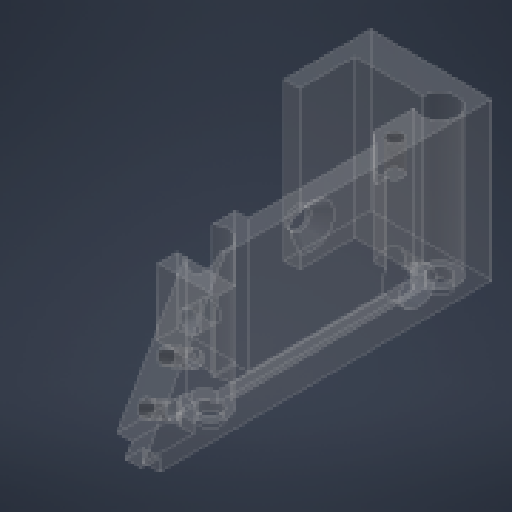
# Autodesk Inventor part: Lewybok
Saved by Autodesk Inventor 2023 (Build 270158000, 158)
## iProperties
Created: 2022-01-30
Part Number: Lewybok
Material: Tworzywo sztuczne PMMA
Document SubType Name: Modeling
Designer: Michał
Density: 1.188 g/cm^3
Appearance: Poliwęglan — przezroczysty
Mass: 9.32104 g
Surface Area: 57.3385 cm^2
Volume: 7.84599 cm^3
Author: Michał
Autodesk Inventor part; units mm, degrees
ref_plane "YZ Plane" through (0, 0, 0) normal (1, 0, 0) x (0, 1, 0)
ref_plane "XZ Plane" through (0, 0, 0) normal (0, 1, 0) x (-1, 0, 0)
ref_plane "XY Plane" through (0, 0, 0) normal (0, 0, 1) x (1, 0, 0)
sketch "Szkic1" plane through (0, 0, 0) normal (0, 1, 0) x (-1, 0, 0)
  line L0 (0, 0) -> (5, 0)
  line L1 (5, 0) -> (5, -58.2)
  line L2 (5, -58.2) -> (0, -58.2)
  line L3 (0, -58.2) -> (0, 0)
  line L4 (5, -58.2) -> (19.35, -58.2)
  line L5 (19.35, -58.2) -> (19.35, -53.2)
  line L6 (19.35, -53.2) -> (5, -53.2)
  line L7 (5, -53.2) -> (5, -58.2)
  line L8 (19.35, -53.2) -> (16.85, -53.2)
  line L9 (16.85, -53.2) -> (16.85, -44.4)
  line L10 (16.85, -44.4) -> (19.35, -44.4)
  line L11 (19.35, -44.4) -> (19.35, -53.2)
  dimension "d0" = 58.2
  dimension "d1" = 5
  dimension "d2" = 19.35
  dimension "d3" = 5
  dimension "d4" = 2.5
  dimension "d5" = 13.8
  constraints: 24 end point, 6 parallel, 3 horizontal, 3 perpendicular
  measures "d0" distance between parallel lines of L2 L0
  measures "d1" distance of L0.start L0.end
  measures "d2" distance between parallel lines of L3 L5
  measures "d3" distance of L4.end L5.end
  measures "d4" distance of L9.end L10.end
  measures "d5" distance between parallel lines of L4 L10
extrude "Wyciągnięcie proste1" add sketch "Szkic1" along normal blind 25
sketch "Szkic2" plane through (0, 0, 0) normal (1, 0, 0) x (0, 0, -1)
  line L0 (0, 0) -> (58.2, 0) projected
  line L1 (0, 0) -> (0, 2)
  line L2 (0, 2) -> (2.3094, 2)
  line L3 (2.3094, 2) -> (15.5885, 25)
  line L4 (53.2, 25) -> (0, 25) projected
  line L5 (15.5885, 25) -> (13.2791, 25)
  line L6 (13.2791, 25) -> (0, 2) construction
  line L7 (0, 2) -> (0, 25)
  line L8 (13.2791, 25) -> (0, 25)
  line L9 (0, 2) -> (5.2, 2)
  line L10 (5.2, 2) -> (5.2, 0)
  dimension "d8" = 5.2
  dimension "d9" = 2
  dimension "d10" = 2
  dimension "d11" = 60
  constraints: 18 end point, 4 point on line, 3 perpendicular, 2 horizontal, 1 parallel, 1 vertical
  measures "d8" distance between parallel lines of L10 L1
  measures "d9" distance between parallel lines of L0 L2
  measures "d10" distance between parallel lines of L3 L6
  measures "d11" angle of L3 L2
extrude "Wyciągnięcie proste2" cut sketch "Szkic2" against normal through all
sketch "Szkic3" plane through (-5, 0, -53.2) normal (-1, 0, 0) x (0, 0, 1)
  line L0 (30.9583, 4.2) -> (33.9583, 4.2)
  line L1 (33.9583, 4.2) -> (33.9583, 14.7)
  line L2 (33.9583, 14.7) -> (30.9583, 14.7)
  line L3 (30.9583, 14.7) -> (30.9583, 4.2)
  line L4 (0, 0) -> (48, 0) projected
  line L5 (33.9583, 14.7) -> (43.5583, 14.7) construction
  line L6 (50.8906, 2) -> (37.6115, 25) construction
  line L7 (33.9583, 4.2) -> (34.2332, 4.2)
  line L8 (34.2332, 4.2) -> (33.9583, 14.7)
  point P0 (53.2, 0)
  dimension "d14" = 4.2
  dimension "d15" = 10.5
  dimension "d16" = 9.6
  dimension "d17" = 3
  dimension "d20" = 88.5
  constraints: 14 end point, 3 horizontal, 2 parallel, 1 perpendicular, 1 point on line
  measures "d14" distance between parallel lines of L4 L0
  measures "d15" distance of L2.end L0.start
  measures "d16" distance of L1.end L5.end
  measures "d17" distance of L0.start L0.end
  measures "d20" angle of L8 L7
extrude "Wyciągnięcie proste3" add sketch "Szkic3" along normal blind 9.3
sketch "Szkic4" plane through (-14.3, 14.7, -19.2417) normal (0, 0.0261769, 0.9996573) x (1, 0, 0)
  line L0 (9.3, -10.5036) -> (0, -10.5036) projected
  line L1 (9.3, 0) -> (9.3, -10.5036) projected
  point P0 (14.3, -15.1987)
  point P1 (5.3, -5.3036)
  dimension "d21" = 5.2
  dimension "d22" = 4
  measures "d21" distance from line of point (5.3, -5.304) L0
  measures "d22" distance from line of L1 point (5.3, -5.304)
hole "Otwór1" at (-9, 9.3982, -19.1029) direction (0, -0.0261769, -0.9996573) diameter 3.4 end up to surface clearance for "Śruba ze łbem stożkowym ISO 2009/7046" size "M3" standard "ISO"
sketch "Szkic5" plane through (-5, 2, -2.3094) normal (0, 0.5, 0.8660254) x (1, 0, 0)
  line L0 (0, 0) -> (5, 0) construction
  line L1 (2.6, 0) -> (2.6, 12.8) construction
  line L2 (5, 26.5581) -> (5, 0) construction
  point P0 (5, -2.8868)
  point P1 (2.6, 6.3)
  dimension "d30" = 2.4
  dimension "d31" = 6.3
  dimension "d32" = 12.8
  constraints: 2 end point, 2 point on line, 1 coincident, 1 vertical
  measures "d30" distance between parallel lines of L2 L1
  measures "d31" distance from line of L0 point (2.6, 6.3)
  measures "d32" distance from line of L0 L1.end
hole "Otwór2" at (-2.4, 7.456, -5.4594) at (-2.4, 13.0851, -8.7094) direction (0, -0.5, -0.8660254) diameter 2.459 depth 5.2 tip angle 118 thread size "M3x0.5" class "6H" standard "ISO Metric profile"
sketch "Szkic8" plane through (0, 0, -58.2) normal (1, 0, 0) x (0, 0, -1)
  line L0 (0, 0) -> (0, 25) projected
  line L1 (-53, 0) -> (0, 0) projected
  point P0 (-58.2, 0)
  point P1 (-11.8, 5)
  dimension "d54" = 11.8
  dimension "d55" = 5
  measures "d54" distance from line of L0 point (-11.8, 5)
  measures "d55" distance from line of L1 point (-11.8, 5)
hole "Otwór4" at (0, 5, -46.4) direction (-1, 0, 0) diameter 3.4 end through all counterbore diameter 5.7 counterbore depth 16.85 clearance for "Śruba ze łbem sześciokątnym wypukłym ISO 24017" size "M3" standard "ISO"
sketch "Szkic6" plane through (0, 25, 0) normal (0, 1, 0) x (1, 0, 0)
  line L0 (0, 15.5885) -> (0, 58.2) construction
  line L1 (0, 58.2) -> (-19.35, 58.2) construction
  point P0 (0, 0)
  point P1 (-3.25, 53.1)
  point P2 (-3.25, 16.5)
  dimension "d40" = 3.25
  dimension "d41" = 5.1
  dimension "d42" = 41.7
  constraints: 1 vertical alignment
  measures "d40" distance from line of L0 point (-3.25, 53.1)
  measures "d41" distance from line of L1 point (-3.25, 53.1)
  measures "d42" distance from line of L1 point (-3.25, 16.5)
hole "Otwór3" at (-3.25, 25, -53.1) at (-3.25, 25, -16.5) direction (0, -1, 0) diameter 3.4 end through all counterbore diameter 5.7 counterbore depth 23.35 clearance for "Śruba ze łbem sześciokątnym wypukłym ISO 24017" size "M3" standard "ISO"
sketch "Szkic9" plane through (-5, 1.65, -18.7494) normal (-1, 0, 0) x (0, 0, 1)
  line L0 (13.5494, 0.35) -> (13.5494, -1.65) construction
  line L1 (13.5494, 0) -> (-34.4506, 0)
  line L2 (-34.4506, 0) -> (-34.4506, 2.2)
  line L3 (-34.4506, 2.2) -> (13.5494, 2.2)
  line L4 (13.5494, 2.2) -> (13.5494, 0)
  line L5 (-34.4506, -1.65) -> (13.5494, -1.65) construction
  line L6 (13.5494, -1.65) -> (-39.4506, -1.65) construction
  line L7 (13.5494, 0) -> (5.5494, 0)
  line L8 (5.5494, 0) -> (5.5494, -1.65)
  line L9 (5.5494, -1.65) -> (13.5494, -1.65)
  line L10 (13.5494, -1.65) -> (13.5494, 0)
  line L11 (-34.4506, -1.65) -> (-34.4506, 23.35) construction
  line L12 (-25.6506, 2.2) -> (-3.4923, 2.2)
  line L13 (-3.4923, 2.2) -> (-3.4923, 23.35)
  line L14 (-3.4923, 23.35) -> (-25.6506, 23.35)
  line L15 (-25.6506, 23.35) -> (-25.6506, 2.2)
  line L16 (-3.4923, 13.05) -> (-3.4923, 2.55) projected
  line L17 (-25.6506, -1.65) -> (-25.6506, 23.35) construction
  line L18 (-32.1011, 23.35) -> (0, 23.35) construction
  line L19 (16.44, 0.35) -> (4.4989, 21.0327) projected
  line L20 (15.3719, 2.2) -> (16.44, 0.35)
  line L21 (16.44, 0.35) -> (13.5494, 0.35)
  line L22 (15.3719, 2.2) -> (13.5494, 2.2)
  line L23 (13.5494, -1.65) -> (13.5494, 0.35) projected
  line L24 (13.5494, 0.35) -> (13.5494, 2.2)
  point P0 (18.7494, -1.65)
  point P1 (-31.4506, -5)
  point P2 (-0.7506, -5)
  dimension "d63" = 1.65
  dimension "d64" = 2.2
  dimension "d65" = 8
  constraints: 32 end point, 7 parallel, 5 collinear, 4 horizontal, 3 perpendicular, 3 point on line, 3 other
  measures "d64" distance between parallel lines of L1 L3
  measures "d65" distance between parallel lines of L0 L8
extrude "Wyciągnięcie proste5" cut sketch "Szkic9" against normal blind 2.4 and the other way blind 11.85 contours L10 L9 L8 L1 | L1 L2 L3 L4 | L4 L22 L19 L21
extrude "Wyciągnięcie proste7" cut sketch "Szkic9" against normal blind 2 contours L3 L15 L14 L13
sketch "Szkic10" plane through (0, 25, 0) normal (0, 1, 0) x (1, 0, 0)
  line L0 (-2.5, 45.2) -> (0, 45.2) construction
  line L1 (0, 15.5885) -> (0, 58.2) construction
  line L2 (-2.5, 45.2) -> (-5, 45.2) construction
  line L3 (-5, 43.7923) -> (-5, 49.0077) construction
  line L4 (0, 58.2) -> (-19.35, 58.2) construction
  circle A0 centre (-2.5, 45.2) radius 2.5
  point P0 (0, 0)
  point P1 (-5, 19.5)
  point P2 (-5, 5.2)
  dimension "d70" = 13
  dimension "d85" = 5
  constraints: 4 end point, 3 point on line, 1 centre point, 1 coincident, 1 collinear, 1 horizontal
  measures "d70" distance from line of L4 L0.start
  measures "d85" diameter of A0
extrude "Wyciągnięcie proste8" add sketch "Szkic10" against normal blind 5.5
hole "Otwór5" at (-2.5, 25, -45.2) direction (0, -1, 0) diameter 2.459 depth 5 thread size "M3x0.5" class "6H" standard "ISO Metric profile"
sketch "Szkic11" plane through (-5, 1.65, -50.8506) normal (-1, 0, 0) x (0, 0, 1)
  line L0 (31.5757, 2.2) -> (31.5757, 0) construction
  line L1 (45.6506, -1.65) -> (-7.3494, -1.65) construction
  line L2 (31.5757, 0) -> (37.1254, 0)
  line L3 (37.1254, 0) -> (37.1254, -1.65)
  line L4 (37.1254, -1.65) -> (31.5757, -1.65)
  line L5 (31.5757, -1.65) -> (31.5757, 0)
  line L6 (37.1254, 0) -> (37.1254, 2.2) projected
  line L7 (0, 0) -> (-2.3494, 0) projected
  line L8 (-2.3494, 0) -> (0, 0)
  line L9 (0, 0) -> (0, -1.65)
  line L10 (0, -1.65) -> (-2.3494, -1.65)
  line L11 (-2.3494, -1.65) -> (-2.3494, 0)
  line L12 (0, 23.35) -> (0, 0) construction
  line L13 (-2.3494, -1.65) -> (37.6506, -1.65) construction
  point P0 (50.8506, -1.65)
  constraints: 16 end point, 4 parallel, 3 collinear, 2 horizontal, 2 perpendicular, 1 point on line
extrude "Wyciągnięcie proste6" add sketch "Szkic11" along normal blind 2
fillet "Zaokrąglenie2" radius 2 3 edges at (-7, 0.825, -50.8506) (-7, 0.825, -19.2749) (-7, 0.825, -13.7251)
chamfer "Faza1" distance 1.936 angle 42.112 1 edges at (-16.85, 5, -44.7) measured on face at (-17.35, 5, -44.7)
equation "\"d59\" = d2 - d4"
equation "\"d67\" = -d1 + d2 - d4"
